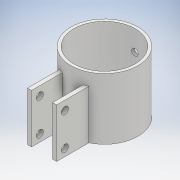
# Autodesk Inventor part: Pok Default Pitch Motor Mount
Saved by Autodesk Inventor 2018.2 (Build 222227000, 227)
## iProperties
Created: 2018-02-12
Part Number: Pok Default Pitch Motor Mount
Material: ABS Plastic
Document SubType Name: Modeling
Designer: Moochster
Density: 1.06 g/cm^3
Appearance: Smooth - White
Author: Moochster
Autodesk Inventor part; units mm, degrees
ref_plane "YZ Plane" through (0, 0, 0) normal (1, 0, 0) x (0, 1, 0)
ref_plane "XZ Plane" through (0, 0, 0) normal (0, 1, 0) x (-1, 0, 0)
ref_plane "XY Plane" through (0, 0, 0) normal (0, 0, 1) x (1, 0, 0)
sketch "Sketch1" plane through (0, 0, 0) normal (0, 0, 1) x (1, 0, 0)
  circle A0 centre (0, 0) radius 15
  circle A1 centre (0, 0) radius 16.4
  line L0 (-7.15, -14.7593) -> (-7.15, -30.5704)
  line L1 (-7.15, -30.5704) -> (-5.15, -30.5704)
  line L2 (-5.15, -30.5704) -> (-5.15, -15.5704)
  line L3 (5.15, -15.5704) -> (5.15, -30.5704)
  line L4 (5.15, -30.5704) -> (7.15, -30.5704)
  line L5 (7.15, -30.5704) -> (7.15, -14.7593)
  dimension "d0" = 1.4
  dimension "d1" = 30
  dimension "d2" = 2
  dimension "d3" = 10.3
  dimension "d4" = 15
  constraints: 12 end point, 4 perpendicular, 4 point on circle, 3 horizontal alignment, 2 centre point, 2 coincident, 2 vertical, 1 collinear
  measures "d0" radial gap between concentric circles of A0 A1
  measures "d1" diameter of A0
  measures "d2" distance of L0.end L1.end
  measures "d3" distance between parallel lines of L3 L2
  measures "d4" distance of L3.start L3.end
extrude "Extrusion1" add sketch "Sketch1" along normal blind 30 contours A1
extrude "Extrusion3" add sketch "Sketch1" along normal blind 24 contours A1 L2 L1 L0 | L5 L4 L3 A1
sketch "Sketch2" plane through (-7.15, -30.5704, 0) normal (-1, 0, 0) x (0, 0, 1)
  circle A0 centre (3.6261, 4) radius 1.75
  circle A1 centre (19.6261, 4) radius 1.75
  line L0 (0, 0) -> (24, 0) projected
  point P0 (0, 30.5704)
  dimension "d7" = 3.5
  dimension "d8" = 3.5
  dimension "d9" = 16
  dimension "d15" = 4
  constraints: 2 centre point, 1 horizontal alignment
  measures "d7" diameter of A0
  measures "d8" diameter of A1
  measures "d9" distance of A0.centre A1.centre
  measures "d15" distance from line of L0 A0.centre
extrude "Extrusion2" cut sketch "Sketch2" against normal through all
sketch "Sketch3" plane through (0, 0, 0) normal (0, 1, 0) x (-1, 0, 0)
  circle A0 centre (0, 8) radius 1.6
  circle A1 centre (0, 20) radius 1.6
  line L0 (15, 0) -> (-15, 0) projected
  point P0 (0, 0)
  point P1 (0, 0)
  dimension "d16" = 3.2
  dimension "d17" = 3.2
  dimension "d18" = 12
  dimension "d19" = 8
  constraints: 2 centre point, 2 vertical alignment, 1 midpoint
  measures "d16" diameter of A0
  measures "d17" diameter of A1
  measures "d18" distance of A1.centre A0.centre
  measures "d19" distance from line of L0 A0.centre
extrude "Extrusion4" cut sketch "Sketch3" along normal through all
body "Solid1"
